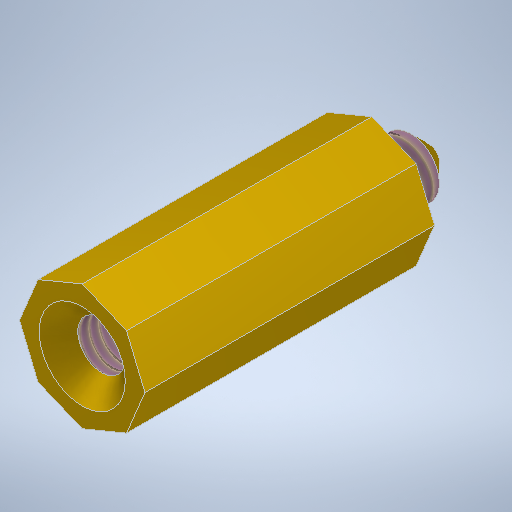
# Autodesk Inventor part: _Supporter
Saved by Autodesk Inventor 2025.1 (Build 291241020, 241B)
## iProperties
Created: 2024-09-22
Part Number: _Supporter
Material: 철, 주조
Document SubType Name: Modeling
Designer: daare
Density: 7.15 g/cm^3
Appearance: 철 회색
Author: daare
Autodesk Inventor part; units mm, degrees
ref_plane "YZ Plane" through (0, 0, 0) normal (1, 0, 0) x (0, 1, 0)
ref_plane "XZ Plane" through (0, 0, 0) normal (0, 1, 0) x (-1, 0, 0)
ref_plane "XY Plane" through (0, 0, 0) normal (0, 0, 1) x (1, 0, 0)
sketch "스케치1" plane through (0, 0, 0) normal (0, 0, 1) x (1, 0, 0)
  line L0 (2.2961, -2.2961) -> (0, -3.2472)
  line L1 (0, -3.2472) -> (-2.2961, -2.2961)
  line L2 (-2.2961, -2.2961) -> (-3.2472, 0)
  line L3 (-3.2472, 0) -> (-2.2961, 2.2961)
  line L4 (-2.2961, 2.2961) -> (0, 3.2472)
  line L5 (0, 3.2472) -> (2.2961, 2.2961)
  line L6 (2.2961, 2.2961) -> (3.2472, 0)
  line L7 (3.2472, 0) -> (2.2961, -2.2961)
  circle A0 centre (0, 0) radius 1.5
  dimension "d0" = 3
  dimension "d1" = 6
  constraints: 16 end point, 2 coincident, 1 centre point, 1 horizontal alignment, 17 other
  measures "d0" diameter of A0
  measures "d1" distance between parallel lines of L2 L6
extrude "돌출1" add sketch "스케치1" along normal blind 15 contours L0 L1 L2 L3 L4 L5 L6 L7 | A0
extrude "돌출2" add sketch "스케치1" against normal blind 3 contours A0
thread "스레드1" size "M3x0.5" class "6g" standard "ISO Metric profile" full length
sketch "스케치2" plane through (0, 0, 15) normal (0, 0, 1) x (1, 0, 0)
  point P0 (0, 0)
  point P1 (0, 0)
  constraints: 1 coincident
hole "구멍1" at (0, 0, 15) direction (0, 0, -1) diameter 2.459 depth 8 tip angle 118 thread size "M3x0.5" class "6H" standard "ISO Metric profile"
chamfer "모따기2" distance 1 angle 45 2 edges at (0, 1.2295, 15) (-1.5, 0, -3)
